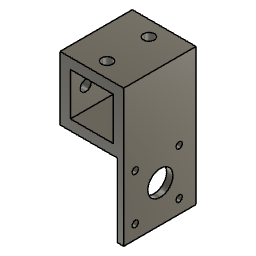
모터브라켓-R (Autodesk Fusion 360 design; units mm, degrees)
Autodesk Fusion 360 part; units mm, degrees
sketch "스케치1" plane through (0, 0, 0) normal (1, 0, 0) x (0, 1, 0)
  line L0 (10.5, 11) -> (-10.5, 11)
  line L1 (-10.5, 11) -> (-10.5, -11)
  line L2 (-10.5, -11) -> (10.5, -11)
  line L3 (10.5, -11) -> (10.5, 11)
  line L4 (10.5, 11) -> (-10.5, -11) construction
  line L5 (-10.5, 11) -> (10.5, -11) construction
  circle A0 centre (10.5, 11) radius 1.5
  circle A1 centre (-10.5, 11) radius 1.5
  circle A2 centre (10.5, -11) radius 1.5
  circle A3 centre (-10.5, -11) radius 1.5
  line L6 (10.5, 0) -> (1.5, 0)
  circle A4 centre (1.5, 0) radius 6
  line L7 (10.5, 0) -> (18.5, 0)
  line L8 (1.5, 0) -> (-16, 0)
  line L9 (18.5, 0) -> (18.5, 17.5)
  line L10 (-16, 0) -> (-16, -17.5)
  line L11 (-16, -17.5) -> (18.5, -17.5)
  line L12 (18.5, -17.5) -> (18.5, 17.5)
  line L13 (18.5, 17.5) -> (-16, 17.5)
  line L14 (-16, 17.5) -> (-16, -17.5)
  line L15 (-16, 17.5) -> (18.5, 17.5)
  line L16 (18.5, 17.5) -> (18.5, 47.9)
  line L17 (18.5, 47.9) -> (-16, 47.9)
  line L18 (-16, 47.9) -> (-16, 17.5)
  dimension "d1" = 21
  dimension "d2" = 22
  dimension "d3" = 3
  dimension "d4" = 3
  dimension "d5" = 3
  dimension "d6" = 3
  dimension "d8" = 9
  dimension "d9" = 12
  dimension "d10" = 8
  dimension "d11" = 17.5
  dimension "d12" = 17.5
  dimension "d13" = 17.5
  dimension "d16" = 30.4
  constraint horizontal L0
  constraint perpendicular L0 L1
  constraint parallel L0 L2
  constraint parallel L1 L3
  constraint coincident L4 origin
  constraint coincident L5 origin
  constraint coincident L0.start L3.end
  constraint coincident L0.end L1.start
  constraint coincident L2.end L3.start
  constraint coincident L1.end L2.start
  constraint midpoint L3 L6.start
  constraint perpendicular L3 L6
  constraint coincident L6.end A4.centre
  constraint perpendicular L3 L7
  constraint perpendicular L1 L8
  constraint perpendicular L7 L9
  constraint perpendicular L8 L10
  constraint horizontal L11
  constraint vertical L12
  constraint horizontal L13
  constraint vertical L14
  constraint horizontal L15
  constraint vertical L16
  constraint horizontal L17
  constraint vertical L18
  measures "d1" distance of L1.end L2.end
  measures "d2" distance of L0.end L1.end
  measures "d3" diameter of A0
  measures "d4" diameter of A1
  measures "d5" diameter of A2
  measures "d6" diameter of A3
  measures "d8" distance of L6.start L6.end
  measures "d9" diameter of A4
  measures "d10" distance of L6.start L7.end
  measures "d11" distance of L6.end L8.end
  measures "d12" distance of L7.end L9.end
  measures "d13" distance of L8.end L10.end
  measures "d16" distance of L13.end L17.end
extrude "돌출1" add sketch "스케치1" along normal blind 3 contours L0 L1 L3 A0 A1 L7 L8 L9 L12 L13 L14 L15 | L0 L1 L3 A0 A1 L6 A4 L8 | L1 L2 L3 A2 A3 L6 A4 L8 | L1 L2 L3 A2 A3 L7 L8 L10 L11 L12 L14 | L13 L15 L16 L17 L18
extrude "돌출2" add sketch "스케치1" against normal blind 27.4 contours L13 L15 L16 L17 L18
sketch "스케치3" plane through (0, 18.5, 0) normal (0, 1, 0) x (-1, 0, 0)
  line L0 (0, -17.5) -> (0, 17.5)
  line L1 (0, 17.5) -> (27.4, 17.5)
  line L2 (27.4, 17.5) -> (27.4, 47.9)
  line L3 (27.4, 47.9) -> (-3, 47.9)
  line L4 (-3, 47.9) -> (-3, -17.5)
  line L5 (-3, -17.5) -> (0, -17.5)
  line L6 (27.4, 17.5) -> (-3, 17.5)
  line L7 (-3, 17.5) -> (-3, 47.9)
  line L8 (-3, 47.9) -> (27.4, 47.9)
  line L9 (27.4, 47.9) -> (27.4, 17.5)
  line L10 (22.4, 42.9) -> (2, 42.9)
  line L11 (2, 42.9) -> (2, 22.5)
  line L12 (2, 22.5) -> (22.4, 22.5)
  line L13 (22.4, 22.5) -> (22.4, 42.9)
  line L14 (22.4, 42.9) -> (2, 22.5) construction
  line L15 (2, 42.9) -> (22.4, 22.5) construction
  point P0 (12.2, 32.7)
  dimension "d23" = 20.4
  dimension "d24" = 20.4
  constraint horizontal L6
  constraint vertical L7
  constraint horizontal L8
  constraint vertical L9
  constraint coincident L3.end L4.start
  constraint coincident L1.end L2.start
  constraint horizontal L10
  constraint perpendicular L10 L11
  constraint parallel L10 L12
  constraint parallel L11 L13
  constraint coincident L14 P0
  constraint coincident L15 P0
  measures "d23" distance of L11.end L12.end
  measures "d24" distance of L10.end L11.end
extrude "돌출4" cut sketch "스케치3" against normal blind 67 contours L10 L11 L12 L13
sketch "스케치4" plane through (0, 0, 47.9) normal (0, 0, 1) x (-1, 0, 0)
  line L0 (27.4, 16) -> (-3, 16)
  line L1 (-3, 16) -> (-3, -18.5)
  line L2 (-3, -18.5) -> (27.4, -18.5)
  line L3 (27.4, -18.5) -> (27.4, 16)
  line L4 (2, -18.5) -> (22.4, -18.5)
  line L5 (22.4, -18.5) -> (22.4, 16)
  line L6 (22.4, 16) -> (2, 16)
  line L7 (2, 16) -> (2, -18.5)
  line L8 (2, -18.5) -> (22.4, 16) construction
  line L9 (22.4, -18.5) -> (2, 16) construction
  line L10 (12.2, -1.25) -> (12.2, 8.75)
  circle A0 centre (12.2, 8.75) radius 2.6
  line L11 (12.2, -1.25) -> (12.2, -11.25)
  circle A1 centre (12.2, -11.25) radius 2.6
  point P0 (12.2, -1.25)
  dimension "d30" = 20.4
  dimension "d31" = 10
  dimension "d32" = 5.2
  dimension "d33" = 10
  dimension "d34" = 5.2
  constraint horizontal L4
  constraint perpendicular L4 L5
  constraint parallel L4 L6
  constraint parallel L5 L7
  constraint coincident L8 P0
  constraint coincident L9 P0
  constraint coincident P0 L10.start
  constraint perpendicular L6 L10
  constraint coincident L10.end A0.centre
  constraint parallel L10 L11
  constraint coincident L11.end A1.centre
  measures "d30" distance of L5.end L6.end
  measures "d31" distance of P0 L10.end
  measures "d32" diameter of A0
  measures "d33" distance of P0 L11.end
  measures "d34" diameter of A1
extrude "돌출6" cut sketch "스케치4" against normal blind 10 contours A0 | A1
sketch "스케치5" plane through (-27.4, 0, 0) normal (-1, 0, 0) x (0, -1, 0)
  line L0 (16, 17.5) -> (16, 47.9)
  line L1 (16, 47.9) -> (-18.5, 47.9)
  line L2 (-18.5, 47.9) -> (-18.5, 17.5)
  line L3 (-18.5, 17.5) -> (16, 17.5)
  line L4 (-18.5, 32.7) -> (-11.25, 32.7)
  circle A0 centre (-11.25, 32.7) radius 2.6
  line L5 (16, 32.7) -> (8.75, 32.7)
  circle A1 centre (8.75, 32.7) radius 2.6
  dimension "d37" = 7.25
  dimension "d38" = 5.2
  dimension "d39" = 7.25
  dimension "d40" = 5.2
  constraint midpoint L2 L4.start
  constraint perpendicular L2 L4
  constraint coincident L4.end A0.centre
  constraint midpoint L0 L5.start
  constraint perpendicular L0 L5
  constraint coincident L5.end A1.centre
  measures "d37" distance of L4.start L4.end
  measures "d38" diameter of A0
  measures "d39" distance of L5.start L5.end
  measures "d40" diameter of A1
extrude "돌출7" cut sketch "스케치5" against normal blind 13 contours A0 | A1
